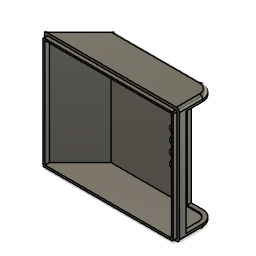
Tapa1_Superior Final (Autodesk Fusion 360 design; units mm, degrees)
Autodesk Fusion 360 part; units mm, degrees
sketch "Boceto1" plane through (0, 0, 0) normal (0, 1, 0) x (1, 0, 0)
  line L0 (0, 0) -> (65, 0)
  line L1 (65, 0) -> (65, 17)
  line L2 (65, 17) -> (0, 17)
  line L3 (0, 17) -> (0, 0)
  line L4 (0, 0) -> (65, 0)
  line L5 (65, 0) -> (65, -2)
  line L6 (65, -2) -> (0, -2)
  line L7 (0, -2) -> (0, 0)
  line L8 (0, 1) -> (16, 17)
  dimension "d1" = 65
  dimension "d2" = 17
  dimension "d5" = 45
  dimension "d6" = 2
  dimension "d17" = 1
  constraint horizontal L0
  constraint vertical L1
  constraint horizontal L2
  constraint vertical L3
  constraint coincident L0.start L3.end
  constraint horizontal L4
  constraint vertical L5
  constraint horizontal L6
  constraint vertical L7
  constraint coincident L3 L8.start
  constraint coincident L2 L8.end
  constraint collinear L1 L5
  measures "d1" distance of L1.end L2.end
  measures "d2" distance of L0.end L1.end
  measures "d5" angle of L3 L8
  measures "d6" distance of L0.start L6.end
  measures "d17" distance of L4 L8.start
extrude "Extruir1" add sketch "Boceto1" along normal blind 56 contours L0 L1 L2 L3 L4 L8 | L0 L4 L5 L6 L7
shell "Vaciado1" thickness 2 removed faces 1 at (43.3333, 18.6667, 2)
sketch "Boceto2" plane through (0, 0, 2) normal (0, 0, 1) x (1, 0, 0)
  line L0 (63, 54) -> (63, 2)
  line L1 (63, 2) -> (2, 2)
  line L2 (2, 2) -> (2, 54)
  line L3 (2, 54) -> (63, 54)
  line L4 (0, 0) -> (65, 0)
  line L5 (65, 0) -> (65, 56)
  line L6 (65, 56) -> (0, 56)
  line L7 (0, 56) -> (0, 0)
  line L8 (0, 0) -> (65, 0)
  line L9 (65, 0) -> (65, 56)
  line L10 (65, 56) -> (0, 56)
  line L11 (0, 56) -> (0, 0)
  line L12 (1, 1) -> (63.8, 1)
  line L13 (63.8, 1) -> (63.8, 54.8)
  line L14 (63.8, 54.8) -> (1, 54.8)
  line L15 (1, 54.8) -> (1, 1)
  dimension "d10" = 1.2
  dimension "d12" = 1.2
  dimension "d13" = 1
  dimension "d14" = 1
  constraint horizontal L8
  constraint vertical L9
  constraint horizontal L10
  constraint vertical L11
  constraint coincident L5.end L6.start
  constraint coincident L4.start L7.end
  constraint horizontal L12
  constraint vertical L13
  constraint horizontal L14
  constraint vertical L15
  measures "d10" distance of L9 L13
  measures "d12" distance of L10 L14
  measures "d13" distance of L8 L12
  measures "d14" distance of L11 L15
extrude "Extruir2" cut sketch "Boceto2" against normal blind 1.8 contours L4 L5 L6 L7 L8 L9 L10 L11
sketch "Boceto3" plane through (0, 0, -17) normal (0, 0, -1) x (-1, 0, 0)
  line L0 (-65, 0) -> (-16, 0)
  line L1 (-16, 0) -> (-16, 56)
  line L2 (-16, 56) -> (-65, 56)
  line L3 (-65, 56) -> (-65, 0)
  line L4 (-65, 53.5) -> (-53.5, 53.5)
  line L5 (-53.5, 53.5) -> (-53.5, 2.5)
  line L6 (-53.5, 2.5) -> (-65, 2.5)
  line L7 (-65, 2.5) -> (-65, 53.5)
  circle A0 centre (-46.8, 15.75) radius 1.75
  circle A1 centre (-46.8, 20.75) radius 1.75
  circle A2 centre (-46.8, 25.75) radius 1.75
  circle A3 centre (-46.8, 30.75) radius 1.75
  circle A4 centre (-46.8, 41) radius 1.75
  dimension "d20" = 2.5
  dimension "d21" = 2.5
  dimension "d22" = 11.5
  dimension "d31" = 3.5
  dimension "d32" = 6.7
  dimension "d33" = 15.75
  dimension "d36" = -15
  dimension "d37" = 0
  dimension "d38" = 3.5
  dimension "d39" = 10.25
  constraint horizontal L4
  constraint vertical L5
  constraint horizontal L6
  constraint vertical L7
  constraint coincident L3 L4.start
  constraint vertical A3.centre A4.centre
  measures "d20" distance of L2 L4
  measures "d21" distance of L0 L6
  measures "d22" distance of L5 L7
  measures "d31" diameter of A0
  measures "d32" distance of L5 A0.centre
  measures "d33" distance of L0 A0.centre
  measures "d38" diameter of A4
  measures "d39" distance of A3.centre A4.centre
extrude "Extruir3" cut sketch "Boceto3" against normal blind 14 contours L3 L4 L5 L6 L7 | A0 | A1 | A2 | A3 | A4
fillet "Empalme2" radius 6 2 edges at (65, 1.25, -17) (65, 54.75, -17)
fillet "Empalme2" radius 4 2 edges at (63, 2.25, -15) (63, 53.75, -15)
fillet "Empalme3" radius 1.5 9 edges at (65, 56, -5.4) (63.2426, 56, -15.2426) (37.5, 56, -17) (16, 28, -17) (8, 56, -9) (65, 0, -5.4) (63.2426, 0, -15.2426) (37.5, 0, -17) (8, 0, -9)
fillet "Empalme3" radius 1.5 1 edges at (0, 28, -1)
fillet "Empalme4" radius 0.5 4 edges at (63.8, 54.8, 1.1) (1, 54.8, 1.1) (63.8, 1, 1.1) (1, 1, 1.1)
equation "d1 = 61 mm + 4 mm"
